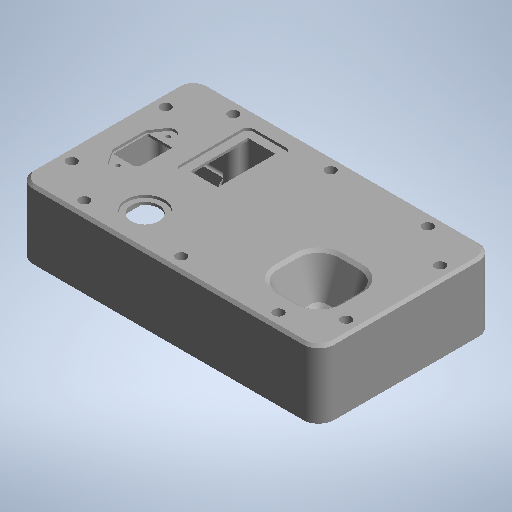
# Autodesk Inventor part: RT_ELE_MC_021_ExtPowerFilterCaseTop
Saved by Autodesk Inventor 2025.4 (Build 294407000, 407)
## iProperties
Created: 2026-08-13
Part Number: RT_ELE_MC_021_ExtPowerFilterCaseTop
Material: Générique
Document SubType Name: Modeling
Designer: louis
Density: 1 g/cm^3
Appearance: Par défaut
Author: louis
Autodesk Inventor part; units mm, degrees
ref_plane "YZ Plane" through (0, 0, 0) normal (1, 0, 0) x (0, 1, 0)
ref_plane "XZ Plane" through (0, 0, 0) normal (0, 1, 0) x (-1, 0, 0)
sketch "Sketch2" plane through (0, 0, 0) normal (0, 0, 1) x (1, 0, 0)
  line L0 (-120, -70) -> (120, -70)
  line L1 (120, -70) -> (120, 70)
  line L2 (120, 70) -> (-120, 70)
  line L3 (-120, 70) -> (-120, -70)
  line L4 (-120, -70) -> (120, 70) construction
  line L5 (120, -70) -> (-120, 70) construction
  line L6 (-112.5, 62.5) -> (112.5, 62.5)
  line L7 (112.5, 62.5) -> (112.5, -62.5)
  line L8 (112.5, -62.5) -> (-112.5, -62.5)
  line L9 (-112.5, -62.5) -> (-112.5, 62.5)
  line L10 (-110, -17.5) -> (110, -17.5) construction
  line L11 (110, -17.5) -> (110, 17.5) construction
  line L12 (110, 17.5) -> (-110, 17.5) construction
  line L13 (-110, 17.5) -> (-110, -17.5) construction
  line L14 (-110, -17.5) -> (110, 17.5) construction
  line L15 (110, -17.5) -> (-110, 17.5) construction
  line L16 (-10, 50) -> (100, 50) construction
  line L17 (100, 50) -> (100, -50) construction
  line L18 (100, -50) -> (-10, -50) construction
  line L19 (-10, -50) -> (-10, 50) construction
  line L20 (-10, 50) -> (100, -50) construction
  line L21 (-10, -50) -> (100, 50) construction
  line L22 (0, 0) -> (110, 0) construction
  circle A0 centre (-109.5, 37.5) radius 2.8
  circle A1 centre (77.5, 59.5) radius 2.8
  circle A2 centre (-77.5, 59.5) radius 2.8
  circle A3 centre (-109.5, -37.5) radius 2.8
  circle A4 centre (-77.5, -59.5) radius 2.8
  circle A5 centre (109.5, 37.5) radius 2.8
  circle A6 centre (109.5, -37.5) radius 2.8
  circle A7 centre (77.5, -59.5) radius 2.8
  line L23 (0, 0) -> (0, 62.5) construction
  circle A8 centre (0, 59.5) radius 2.8
  circle A9 centre (0, -59.5) radius 2.8
  circle A10 centre (-77.5, 59.5) radius 6
  circle A11 centre (77.5, 59.5) radius 6
  circle A12 centre (0, 59.5) radius 6
  circle A13 centre (-109.5, 37.5) radius 6
  circle A14 centre (109.5, 37.5) radius 6
  circle A15 centre (-109.5, -37.5) radius 6
  circle A16 centre (-77.5, -59.5) radius 6
  circle A17 centre (0, -59.5) radius 6
  circle A18 centre (77.5, -59.5) radius 6
  circle A19 centre (109.5, -37.5) radius 6
  point P0 (100, 0)
  point P1 (-112.5, 42.6962)
  point P2 (-82.6962, 62.5)
  point P3 (-72.3038, 62.5)
  point P4 (-5.1962, 62.5)
  point P5 (5.1962, 62.5)
  point P6 (72.3038, 62.5)
  point P7 (82.6962, 62.5)
  point P8 (112.5, 42.6962)
  point P9 (112.5, 32.3038)
  point P10 (112.5, -32.3038)
  point P11 (112.5, -42.6962)
  point P12 (82.6962, -62.5)
  point P13 (72.3038, -62.5)
  point P14 (5.1962, -62.5)
  point P15 (-5.1962, -62.5)
  point P16 (-72.3038, -62.5)
  point P17 (-82.6962, -62.5)
  point P18 (-112.5, -42.6962)
  point P19 (-112.5, -32.3038)
  point P20 (-112.5, 32.3038)
  dimension "d0" = 240
  dimension "d1" = 140
  dimension "d2" = 7.5
  dimension "d3" = 220
  dimension "d4" = 35
  dimension "d5" = 110
  dimension "d6" = 100
  dimension "d7" = 10
  dimension "d8" = 5.6
  dimension "d9" = 5.6
  dimension "d10" = 3
  dimension "d11" = 3
  dimension "d12" = 5.6
  dimension "d13" = 3
  dimension "d14" = 25
  dimension "d15" = 35
  dimension "d16" = 12
  dimension "d17" = 12
  dimension "d18" = 12
  dimension "d19" = 12
  dimension "d20" = 12
  constraints: 48 end point, 20 centre point, 8 parallel, 7 midpoint, 5 coincident, 5 symmetric about line, 4 perpendicular, 3 horizontal, 2 point on line, 15 other
  measures "d0" distance of L5.end L4.end
  measures "d1" distance of L4.end L0.end
  measures "d2" distance between parallel lines of L2 L6
  measures "d3" distance of L15.end L12.start
  measures "d4" distance of L12.start L15.start
  measures "d5" distance of L20.end L19.start
  measures "d6" distance of L16.end L20.end
  measures "d7" distance from line of point (100, 0) L11
  measures "d8" diameter of A0
  measures "d9" diameter of A2
  measures "d10" distance from line of L6 A2.centre
  measures "d11" distance from line of L9 A0.centre
  measures "d12" diameter of A8
  measures "d13" distance from line of L6 A8.centre
  measures "d14" distance from line of L6 A0.centre
  measures "d15" distance from line of L9 A2.centre
  measures "d16" diameter of A13
  measures "d17" diameter of A10
  measures "d18" diameter of A11
  measures "d19" diameter of A12
  measures "d20" diameter of A14
extrude "Extrusion2" add sketch "Sketch2" against normal blind 4 contours L3 L2 L1 L0 | L6 A10 A12 A11 L7 A14 A19 L8 A18 A17 A16 L9 A15 A13 | A10 L6 | L6 A10 | A13 L9 | L9 A13 | A12 L6 | L6 A12 | A15 L9 | L9 A15 | A11 L6 | L6 A11 | A16 L8 | L8 A16 | A14 L7 | L7 A14 | A17 L8 | L8 A17 | A19 L7 | L7 A19 | A18 L8 | L8 A18 | A0 | A1 | A2 | A3 | A4 | A5 | A6 | A7 | A8 | A9
extrude "Extrusion1" add sketch "Sketch2" against normal blind 54 contours L3 L2 L1 L0 | A10 L6 | L6 A10 | A13 L9 | L9 A13 | A12 L6 | L6 A12 | A15 L9 | L9 A15 | A11 L6 | L6 A11 | A16 L8 | L8 A16 | A14 L7 | L7 A14 | A17 L8 | L8 A17 | A19 L7 | L7 A19 | A18 L8 | L8 A18 | A0 | A1 | A2 | A3 | A4 | A5 | A6 | A7 | A8 | A9
fillet "Fillet2" radius 12.5 4 edges at (-120, 70, -27) (120, 70, -27) (-120, -70, -27) (120, -70, -27)
fillet "Fillet3" radius 5 4 edges at (-112.5, 62.5, -29) (-112.5, -62.5, -29) (112.5, 62.5, -29) (112.5, -62.5, -29)
chamfer "Chamfer1" distance 2 angle 45 26 edges at (-38.75, -62.5, -4) (-95.0981, -62.5, -4) (-111.0355, -61.0355, -4) (-112.5, -50.0981, -4) (-112.5, 0, -4) (38.75, -62.5, -4) (95.0981, -62.5, -4) (111.0355, -61.0355, -4) (112.5, -50.0981, -4) (112.5, 0, -4) (95.0981, 62.5, -4) (111.0355, 61.0355, -4) (112.5, 50.0981, -4) (38.75, 62.5, -4) (-38.75, 62.5, -4) (-95.0981, 62.5, -4) (-111.0355, 61.0355, -4) (-112.5, 50.0981, -4) (0, 70, 0) (-116.3388, 66.3388, 0) (-120, 0, 0) (-116.3388, -66.3388, 0) (0, -70, 0) (116.3388, -66.3388, 0) (120, 0, 0) (116.3388, 66.3388, 0)
fillet "Fillet1" radius 5 30 edges at (-112.5, -42.6962, -30) (-82.6962, -62.5, -30) (-72.3038, -62.5, -30) (-5.1962, -62.5, -30) (5.1962, -62.5, -30) (72.3038, -62.5, -30) (82.6962, -62.5, -30) (112.5, -42.6962, -30) (112.5, -32.3038, -30) (112.5, 32.3038, -30) (112.5, 42.6962, -30) (82.6962, 62.5, -30) (72.3038, 62.5, -30) (5.1962, 62.5, -30) (-5.1962, 62.5, -30) (-72.3038, 62.5, -30) (-82.6962, 62.5, -30) (-112.5, 32.3038, -30) (-112.5, 42.6962, -30) (-112.5, -32.3038, -30) (-77.5, -53.5, -4) (-103.5, -37.5, -4) (0, 53.5, -4) (-77.5, 53.5, -4) (103.5, 37.5, -4) (77.5, 53.5, -4) (-103.5, 37.5, -4) (0, -53.5, -4) (77.5, -53.5, -4) (103.5, -37.5, -4)
hole "Hole1" at (77.5, -59.5, 0) at (109.5, -37.5, 0) at (109.5, 37.5, 0) at (77.5, 59.5, 0) at (0, 59.5, 0) at (-77.5, 59.5, 0) at (-109.5, 37.5, 0) at (-109.5, -37.5, 0) at (-77.5, -59.5, 0) at (0, -59.5, 0) direction (0, 0, -1) diameter 4.5 end through all counterbore diameter 8 counterbore depth 44 clearance for "Socket Head Cap Screw" size "M4" standard "Ansi Metric M Profile"
sketch "Sketch3" plane through (0, 0, 0) normal (0, 0, 1) x (1, 0, 0)
  line L0 (-35.25, 50.8) -> (-57.25, 50.8)
  line L1 (-57.25, 50.8) -> (-57.25, 4.8)
  line L2 (-57.25, 4.8) -> (-35.25, 4.8)
  line L3 (-35.25, 4.8) -> (-35.25, 50.8)
  line L4 (-35.25, 50.8) -> (-57.25, 4.8) construction
  line L5 (-57.25, 50.8) -> (-35.25, 4.8) construction
  line L6 (-33.75, -1.7) -> (-58.75, -1.7)
  line L7 (-63.75, 3.3) -> (-63.75, 52.3)
  line L8 (-58.75, 57.3) -> (-33.75, 57.3)
  line L9 (-28.75, 52.3) -> (-28.75, 3.3)
  arc A0 (-33.75, -1.7) -> (-28.75, 3.3) centre (-33.75, 3.3) ccw
  arc A1 (-28.75, 52.3) -> (-33.75, 57.3) centre (-33.75, 52.3) ccw
  arc A2 (-58.75, 57.3) -> (-63.75, 52.3) centre (-58.75, 52.3) ccw
  arc A3 (-63.75, 3.3) -> (-58.75, -1.7) centre (-58.75, 3.3) ccw
  circle A4 centre (-90, 20) radius 5.6
  circle A5 centre (-90, -20) radius 5.6
  line L10 (-101.25, -12.25) -> (-101.25, 12.25)
  line L11 (-98.25, 15.25) -> (-81.75, 15.25)
  line L12 (-78.75, 12.25) -> (-78.75, -12.25)
  line L13 (-81.75, -15.25) -> (-98.25, -15.25)
  line L14 (-101.25, -15.25) -> (-78.75, 15.25) construction
  line L15 (-101.25, 15.25) -> (-78.75, -15.25) construction
  line L16 (-109.6425, -25.6) -> (-109.6425, 25.6) construction
  line L17 (-109.6425, 25.6) -> (-70.3575, 25.6) construction
  line L18 (-70.3575, 25.6) -> (-70.3575, -25.6) construction
  line L19 (-70.3575, -25.6) -> (-109.6425, -25.6) construction
  line L20 (-109.6425, -25.6) -> (-70.3575, 25.6) construction
  line L21 (-109.6425, 25.6) -> (-70.3575, -25.6) construction
  line L22 (-90, 20) -> (-90, 0) construction
  arc A6 (-78.75, 12.25) -> (-81.75, 15.25) centre (-81.75, 12.25) ccw
  arc A7 (-81.75, -15.25) -> (-78.75, -12.25) centre (-81.75, -12.25) ccw
  arc A8 (-101.25, -12.25) -> (-98.25, -15.25) centre (-98.25, -12.25) ccw
  arc A9 (-98.25, 15.25) -> (-101.25, 12.25) centre (-98.25, 12.25) ccw
  line L23 (-85.3308, 23.0917) -> (-79.2487, 13.9063)
  line L24 (-94.6692, 23.0917) -> (-100.7513, 13.9063)
  line L25 (-94.6692, -23.0917) -> (-100.7513, -13.9063)
  line L26 (-79.2487, -13.9063) -> (-85.3308, -23.0917)
  line L27 (-90, 0) -> (-90, -20) construction
  line L28 (-100, -14) -> (-100, 14)
  line L29 (-100, 14) -> (-80, 14)
  line L30 (-80, 14) -> (-80, -14)
  line L31 (-80, -14) -> (-100, -14)
  line L32 (-100, -14) -> (-80, 14) construction
  line L33 (-100, 14) -> (-80, -14) construction
  circle A10 centre (-46.25, -42.2) radius 11
  circle A11 centre (-46.25, -42.2) radius 15.1
  line L34 (-46.25, 27.8) -> (-46.25, -42.2) construction
  line L35 (-101.25, 57.3) -> (-28.75, 57.3)
  line L36 (-28.75, 57.3) -> (-28.75, -57.3)
  line L37 (-28.75, -57.3) -> (-101.25, -57.3)
  line L38 (-101.25, -57.3) -> (-101.25, 57.3)
  line L39 (-101.25, 57.3) -> (-28.75, -57.3) construction
  line L40 (-28.75, 57.3) -> (-101.25, -57.3) construction
  line L41 (-65, 0) -> (-90, 0) construction
  line L42 (0, 0) -> (-65, 0) construction
  point P0 (-28.75, -1.7)
  point P1 (-63.75, -1.7)
  dimension "d38" = 22
  dimension "d39" = 46
  dimension "d40" = 35
  dimension "d41" = 5
  dimension "d42" = 22.5
  dimension "d43" = 30.5
  dimension "d45" = 51.2
  dimension "d46" = 3
  dimension "d47" = 28
  dimension "d48" = 20
  dimension "d49" = 22
  dimension "d50" = 30.2
  dimension "d51" = 70
  dimension "d54" = 40
  dimension "d55" = 25
  dimension "d56" = 65
  constraints: 86 end point, 27 tangent, 24 point on circle, 14 parallel, 12 centre point, 12 point on line, 10 midpoint, 7 equal radius, 7 perpendicular, 4 collinear, 4 horizontal, 1 coincident, 1 vertical, 3 other
  measures "d38" distance of L2.end L1.end
  measures "d39" distance of L1.end L0.end
  measures "d40" distance of point (-28.75, -1.7) point (-63.75, -1.7)
  measures "d41" radius of A0
  measures "d42" distance of L15.end L14.start
  measures "d43" distance of L14.end L15.end
  measures "d45" distance of L17.end L18.end
  measures "d46" radius of A6
  measures "d47" distance of L29.end L30.end
  measures "d48" distance of L28.end L29.end
  measures "d49" diameter of A10
  measures "d50" diameter of A11
  measures "d51" distance of L34.start L34.end
  measures "d54" distance of L22.start L27.end
  measures "d55" distance of L41.start L22.end
  measures "d56" distance of L42.start L41.start
extrude "Extrusion3" cut sketch "Sketch3" against normal through all contours L3 L2 L1 L0 | L28 L29 L30 L31 | A10
extrude "Extrusion4" cut sketch "Sketch3" against normal blind 2 contours L3 L2 L1 L0 | A11 | L6 A3 L7 A2 L8 A1 L9 A0 | L10 A9 L11 A4 A6 L12 A7 L13 A5 A8 | A8 L13 A5 L25 | L24 A4 L11 A9 | A5 L13 | A4 L11 | A5 L13 | A5 L13 A7 L26 | L11 A4 | L23 A6 L11 A4 | L28 L29 L30 L31 | A10
hole "Hole2" at (-90, 20, 0) at (-90, -20, 0) direction (0, 0, -1) diameter 3.3 end through all
fillet "Fillet4" radius 1 8 edges at (-57.25, 50.8, -3) (-57.25, 4.8, -3) (-35.25, 4.8, -3) (-35.25, 50.8, -3) (-80, 14, -3) (-100, 14, -3) (-100, -14, -3) (-80, -14, -3)
ref_plane "Work Plane1" through (0, 0, -34) normal (0, 0, -1) x (-1, 0, 0)
sketch "Sketch4" plane through (0, 0, -34) normal (0, 0, -1) x (-1, 0, 0)
  line L0 (-62, -30) -> (-78, -30)
  line L1 (-80, -28) -> (-80, -12)
  line L2 (-78, -10) -> (-62, -10)
  line L3 (-60, -12) -> (-60, -28)
  line L4 (-60, -30) -> (-80, -10) construction
  line L5 (-80, -30) -> (-60, -10) construction
  line L6 (-82.5, 0) -> (-57.5, 0)
  line L7 (-50, -7.5) -> (-50, -32.5)
  line L8 (-57.5, -40) -> (-82.5, -40)
  line L9 (-90, -32.5) -> (-90, -7.5)
  line L10 (-90, 0) -> (-50, -40) construction
  line L11 (-50, 0) -> (-90, -40) construction
  arc A0 (-62, -30) -> (-60, -28) centre (-62, -28) ccw
  arc A1 (-60, -12) -> (-62, -10) centre (-62, -12) ccw
  arc A2 (-78, -10) -> (-80, -12) centre (-78, -12) ccw
  arc A3 (-80, -28) -> (-78, -30) centre (-78, -28) ccw
  arc A4 (-57.5, -40) -> (-50, -32.5) centre (-57.5, -32.5) ccw
  arc A5 (-90, -32.5) -> (-82.5, -40) centre (-82.5, -32.5) ccw
  arc A6 (-82.5, 0) -> (-90, -7.5) centre (-82.5, -7.5) ccw
  arc A7 (-50, -7.5) -> (-57.5, 0) centre (-57.5, -7.5) ccw
  line L12 (-112.5, -26.6833) -> (-112.5, 26.6833) projected
  line L13 (-78, -32.5) -> (-62, -32.5)
  arc A8 (-62, -32.5) -> (-57.5, -28) centre (-62, -28) ccw
  line L14 (-57.5, -28) -> (-57.5, -12)
  arc A9 (-57.5, -12) -> (-62, -7.5) centre (-62, -12) ccw
  line L15 (-62, -7.5) -> (-78, -7.5)
  arc A10 (-78, -7.5) -> (-82.5, -12) centre (-78, -12) ccw
  line L16 (-82.5, -12) -> (-82.5, -28)
  arc A11 (-82.5, -28) -> (-78, -32.5) centre (-78, -28) ccw
  point P0 (0, 0)
  point P1 (-70, -20)
  dimension "d70" = 20
  dimension "d71" = 20
  dimension "d72" = 40
  dimension "d73" = 40
  dimension "d74" = 2
  dimension "d75" = 7.5
  dimension "d76" = 20
  dimension "d77" = 70
  dimension "d78" = 22.5
  dimension "d89" = 2.5
  constraints: 32 end point, 24 point on circle, 16 point on line, 16 tangent, 12 centre point, 6 equal radius, 6 parallel, 4 midpoint, 3 perpendicular, 2 horizontal, 7 other
  measures "d70" distance of L4.end L5.end
  measures "d71" distance of L5.start L4.end
  measures "d72" distance of L10.end L11.end
  measures "d73" distance of L11.start L10.end
  measures "d74" radius of A0
  measures "d75" radius of A4
  measures "d76" vertical distance of point (0, 0) point (-70, -20)
  measures "d77" horizontal distance of point (-70, -20) point (0, 0)
  measures "d78" distance between parallel lines of L12 L9
  measures "d89" distance between parallel lines of L0 L13
sketch "Sketch5" plane through (0, 0, 0) normal (0, 0, 1) x (1, 0, 0)
  line L0 (62, -30) -> (78, -30) construction
  line L1 (78, -10) -> (62, -10) construction
  line L2 (60, -30) -> (80, -10) construction
  line L3 (80, -30) -> (60, -10) construction
  line L4 (57.5, -40) -> (82.5, -40) construction
  line L5 (82.5, 0) -> (57.5, 0) construction
  line L6 (50, 0) -> (90, -40) construction
  arc A0 (62, -10) -> (60, -12) centre (62, -12) ccw construction
  line L7 (50, -7.5) -> (50, -32.5) construction
  arc A1 (57.5, 0) -> (50, -7.5) centre (57.5, -7.5) ccw construction
  line L8 (60, -12) -> (60, -28) construction
  arc A2 (80, -12) -> (78, -10) centre (78, -12) ccw construction
  arc A3 (78, -30) -> (80, -28) centre (78, -28) ccw construction
  line L9 (80, -28) -> (80, -12) construction
  arc A4 (82.5, -40) -> (90, -32.5) centre (82.5, -32.5) ccw construction
  line L10 (90, -32.5) -> (90, -7.5) construction
  arc A5 (90, -7.5) -> (82.5, 0) centre (82.5, -7.5) ccw construction
  arc A6 (50, -32.5) -> (57.5, -40) centre (57.5, -32.5) ccw construction
  arc A7 (60, -28) -> (62, -30) centre (62, -28) ccw construction
  line L11 (37.5, -7.5) -> (37.5, -32.5)
  arc A8 (37.5, -32.5) -> (57.5, -52.5) centre (57.5, -32.5) ccw
  line L12 (57.5, -52.5) -> (82.5, -52.5)
  arc A9 (82.5, -52.5) -> (102.5, -32.5) centre (82.5, -32.5) ccw
  line L13 (102.5, -32.5) -> (102.5, -7.5)
  arc A10 (102.5, -7.5) -> (82.5, 12.5) centre (82.5, -7.5) ccw
  line L14 (82.5, 12.5) -> (57.5, 12.5)
  arc A11 (57.5, 12.5) -> (37.5, -7.5) centre (57.5, -7.5) ccw
  line L15 (47.5, -28) -> (47.5, -12)
  arc A12 (62, 2.5) -> (47.5, -12) centre (62, -12) ccw
  line L16 (62, 2.5) -> (78, 2.5)
  arc A13 (92.5, -12) -> (78, 2.5) centre (78, -12) ccw
  line L17 (92.5, -12) -> (92.5, -28)
  arc A14 (78, -42.5) -> (92.5, -28) centre (78, -28) ccw
  line L18 (78, -42.5) -> (62, -42.5)
  arc A15 (47.5, -28) -> (62, -42.5) centre (62, -28) ccw
  line L19 (62, -45) -> (78, -45)
  arc A16 (78, -45) -> (95, -28) centre (78, -28) ccw
  line L20 (95, -28) -> (95, -12)
  arc A17 (95, -12) -> (78, 5) centre (78, -12) ccw
  line L21 (78, 5) -> (62, 5)
  arc A18 (62, 5) -> (45, -12) centre (62, -12) ccw
  line L22 (45, -12) -> (45, -28)
  arc A19 (45, -28) -> (62, -45) centre (62, -28) ccw
  point P0 (0, 0)
  point P1 (70, -20)
  point P2 (50, -40)
  dimension "d79" = 12.5
  dimension "d80" = 12.5
  dimension "d90" = 2.5
  constraints: 24 end point, 24 point on circle, 12 centre point, 21 other
  measures "d79" radial gap between concentric circles of A1 A11
  measures "d80" distance between parallel lines of L8 L15
  measures "d90" distance between parallel lines of L18 L19
loft "Loft1" add profiles "Sketch4", "Sketch5" contours L0 A3 L1 A2 L2 A1 L3 A0 | L6 A7 L7 A4 L8 A5 L9 A6 | A11 L16 A10 L15 A9 L14 A8 L13 / A11 L14 A10 L13 A9 L12 A8 L11 | L15 A12 L16 A13 L17 A14 L18 A15 | A19 L22 A18 L21 A17 L20 A16 L19
loft "Loft2" cut profiles "Sketch4", "Sketch5" contours L0 A3 L1 A2 L2 A1 L3 A0 | A11 L16 A10 L15 A9 L14 A8 L13 / L15 A12 L16 A13 L17 A14 L18 A15 | A19 L22 A18 L21 A17 L20 A16 L19
extrude "Extrusion5" add sketch "Sketch4" against normal blind 2 contours L6 A7 L7 A4 L8 A5 L9 A6 | A11 L16 A10 L15 A9 L14 A8 L13
chamfer "Chamfer2" distance 3.2 angle 45 8 edges at (58.2981, -8.2981, -32) (70, -6.7647, -32) (81.7019, -8.2981, -32) (83.2353, -20, -32) (81.7019, -31.7019, -32) (70, -33.2353, -32) (58.2981, -31.7019, -32) (56.7647, -20, -32)
chamfer "Chamfer3" distance 2 angle 45 8 edges at (49.9792, 0.0208, 0) (70, 5, 0) (90.0208, 0.0208, 0) (95, -20, 0) (90.0208, -40.0208, 0) (70, -45, 0) (49.9792, -40.0208, 0) (45, -20, 0)
chamfer "Chamfer4" distance 1 angle 45 10 edges at (77.5, 63.5, -44) (109.5, 41.5, -44) (0, 63.5, -44) (-77.5, 63.5, -44) (-109.5, 41.5, -44) (-109.5, -33.5, -44) (-77.5, -55.5, -44) (0, -55.5, -44) (77.5, -55.5, -44) (109.5, -33.5, -44)
sketch "Sketch6" plane through (0, 0, -54) normal (0, 0, -1) x (-1, 0, 0)
  circle A0 centre (0, -59.5) radius 2.25 projected
  circle A1 centre (77.5, -59.5) radius 2.25 projected
  circle A2 centre (109.5, -37.5) radius 2.25 projected
  circle A3 centre (109.5, 37.5) radius 2.25 projected
  circle A4 centre (77.5, 59.5) radius 2.25 projected
  circle A5 centre (0, 59.5) radius 2.25 projected
  circle A6 centre (-77.5, 59.5) radius 2.25 projected
  circle A7 centre (-109.5, 37.5) radius 2.25 projected
  circle A8 centre (-109.5, -37.5) radius 2.25 projected
  circle A9 centre (-77.5, -59.5) radius 2.25 projected
  arc A10 (-120, -57.5) -> (-107.5, -70) centre (-107.5, -57.5) ccw projected
  line L0 (-107.5, -70) -> (107.5, -70) projected
  arc A11 (107.5, -70) -> (120, -57.5) centre (107.5, -57.5) ccw projected
  line L1 (120, -57.5) -> (120, 57.5) projected
  arc A12 (120, 57.5) -> (107.5, 70) centre (107.5, 57.5) ccw projected
  line L2 (107.5, 70) -> (-107.5, 70) projected
  arc A13 (-107.5, 70) -> (-120, 57.5) centre (-107.5, 57.5) ccw projected
  line L3 (-120, 57.5) -> (-120, -57.5) projected
  arc A14 (108.4091, 43.4) -> (108.4091, 31.6) centre (109.5, 37.5) ccw projected
  arc A15 (112.5, 26.6833) -> (108.4091, 31.6) centre (107.5, 26.6833) ccw projected
  line L4 (112.5, 26.6833) -> (112.5, -26.6833) projected
  arc A16 (108.4091, -31.6) -> (112.5, -26.6833) centre (107.5, -26.6833) ccw projected
  arc A17 (108.4091, -31.6) -> (108.4091, -43.4) centre (109.5, -37.5) ccw projected
  arc A18 (112.5, -48.3167) -> (108.4091, -43.4) centre (107.5, -48.3167) ccw projected
  line L5 (112.5, -48.3167) -> (112.5, -57.5) projected
  arc A19 (107.5, -62.5) -> (112.5, -57.5) centre (107.5, -57.5) ccw projected
  line L6 (107.5, -62.5) -> (88.3167, -62.5) projected
  arc A20 (83.4, -58.4091) -> (88.3167, -62.5) centre (88.3167, -57.5) ccw projected
  arc A21 (83.4, -58.4091) -> (71.6, -58.4091) centre (77.5, -59.5) ccw projected
  arc A22 (66.6833, -62.5) -> (71.6, -58.4091) centre (66.6833, -57.5) ccw projected
  line L7 (66.6833, -62.5) -> (10.8167, -62.5) projected
  arc A23 (5.9, -58.4091) -> (10.8167, -62.5) centre (10.8167, -57.5) ccw projected
  arc A24 (5.9, -58.4091) -> (-5.9, -58.4091) centre (0, -59.5) ccw projected
  arc A25 (-10.8167, -62.5) -> (-5.9, -58.4091) centre (-10.8167, -57.5) ccw projected
  line L8 (-10.8167, -62.5) -> (-66.6833, -62.5) projected
  arc A26 (-71.6, -58.4091) -> (-66.6833, -62.5) centre (-66.6833, -57.5) ccw projected
  arc A27 (-71.6, -58.4091) -> (-83.4, -58.4091) centre (-77.5, -59.5) ccw projected
  arc A28 (-88.3167, -62.5) -> (-83.4, -58.4091) centre (-88.3167, -57.5) ccw projected
  line L9 (-88.3167, -62.5) -> (-107.5, -62.5) projected
  arc A29 (-112.5, -57.5) -> (-107.5, -62.5) centre (-107.5, -57.5) ccw projected
  line L10 (-112.5, -57.5) -> (-112.5, -48.3167) projected
  arc A30 (-108.4091, -43.4) -> (-112.5, -48.3167) centre (-107.5, -48.3167) ccw projected
  arc A31 (-108.4091, -43.4) -> (-108.4091, -31.6) centre (-109.5, -37.5) ccw projected
  arc A32 (-112.5, -26.6833) -> (-108.4091, -31.6) centre (-107.5, -26.6833) ccw projected
  line L11 (-112.5, -26.6833) -> (-112.5, 26.6833) projected
  arc A33 (-108.4091, 31.6) -> (-112.5, 26.6833) centre (-107.5, 26.6833) ccw projected
  arc A34 (-108.4091, 31.6) -> (-108.4091, 43.4) centre (-109.5, 37.5) ccw projected
  arc A35 (-112.5, 48.3167) -> (-108.4091, 43.4) centre (-107.5, 48.3167) ccw projected
  line L12 (-112.5, 48.3167) -> (-112.5, 57.5) projected
  arc A36 (-107.5, 62.5) -> (-112.5, 57.5) centre (-107.5, 57.5) ccw projected
  line L13 (-107.5, 62.5) -> (-88.3167, 62.5) projected
  arc A37 (-83.4, 58.4091) -> (-88.3167, 62.5) centre (-88.3167, 57.5) ccw projected
  arc A38 (-83.4, 58.4091) -> (-71.6, 58.4091) centre (-77.5, 59.5) ccw projected
  arc A39 (-66.6833, 62.5) -> (-71.6, 58.4091) centre (-66.6833, 57.5) ccw projected
  line L14 (-66.6833, 62.5) -> (-10.8167, 62.5) projected
  arc A40 (-5.9, 58.4091) -> (-10.8167, 62.5) centre (-10.8167, 57.5) ccw projected
  arc A41 (-5.9, 58.4091) -> (5.9, 58.4091) centre (0, 59.5) ccw projected
  arc A42 (10.8167, 62.5) -> (5.9, 58.4091) centre (10.8167, 57.5) ccw projected
  line L15 (10.8167, 62.5) -> (66.6833, 62.5) projected
  arc A43 (71.6, 58.4091) -> (66.6833, 62.5) centre (66.6833, 57.5) ccw projected
  arc A44 (71.6, 58.4091) -> (83.4, 58.4091) centre (77.5, 59.5) ccw projected
  arc A45 (88.3167, 62.5) -> (83.4, 58.4091) centre (88.3167, 57.5) ccw projected
  line L16 (88.3167, 62.5) -> (107.5, 62.5) projected
  arc A46 (112.5, 57.5) -> (107.5, 62.5) centre (107.5, 57.5) ccw projected
  line L17 (112.5, 57.5) -> (112.5, 48.3167) projected
  arc A47 (108.4091, 43.4) -> (112.5, 48.3167) centre (107.5, 48.3167) ccw projected
  arc A48 (-69.6333, -58.0455) -> (-85.3667, -58.0455) centre (-77.5, -59.5) ccw
  arc A49 (-69.6333, -58.0455) -> (-66.6833, -60.5) centre (-66.6833, -57.5) ccw
  line L18 (-66.6833, -60.5) -> (-10.8167, -60.5)
  arc A50 (-10.8167, -60.5) -> (-7.8667, -58.0455) centre (-10.8167, -57.5) ccw
  arc A51 (7.8667, -58.0455) -> (-7.8667, -58.0455) centre (0, -59.5) ccw
  arc A52 (7.8667, -58.0455) -> (10.8167, -60.5) centre (10.8167, -57.5) ccw
  line L19 (10.8167, -60.5) -> (66.6833, -60.5)
  arc A53 (66.6833, -60.5) -> (69.6333, -58.0455) centre (66.6833, -57.5) ccw
  arc A54 (85.3667, -58.0455) -> (69.6333, -58.0455) centre (77.5, -59.5) ccw
  arc A55 (85.3667, -58.0455) -> (88.3167, -60.5) centre (88.3167, -57.5) ccw
  line L20 (88.3167, -60.5) -> (107.5, -60.5)
  arc A56 (107.5, -60.5) -> (110.5, -57.5) centre (107.5, -57.5) ccw
  line L21 (110.5, -57.5) -> (110.5, -48.3167)
  arc A57 (110.5, -48.3167) -> (108.0455, -45.3667) centre (107.5, -48.3167) ccw
  arc A58 (108.0455, -29.6333) -> (108.0455, -45.3667) centre (109.5, -37.5) ccw
  arc A59 (108.0455, -29.6333) -> (110.5, -26.6833) centre (107.5, -26.6833) ccw
  line L22 (110.5, -26.6833) -> (110.5, 26.6833)
  arc A60 (110.5, 26.6833) -> (108.0455, 29.6333) centre (107.5, 26.6833) ccw
  arc A61 (108.0455, 45.3667) -> (108.0455, 29.6333) centre (109.5, 37.5) ccw
  arc A62 (108.0455, 45.3667) -> (110.5, 48.3167) centre (107.5, 48.3167) ccw
  line L23 (110.5, 48.3167) -> (110.5, 57.5)
  arc A63 (110.5, 57.5) -> (107.5, 60.5) centre (107.5, 57.5) ccw
  line L24 (107.5, 60.5) -> (88.3167, 60.5)
  arc A64 (88.3167, 60.5) -> (85.3667, 58.0455) centre (88.3167, 57.5) ccw
  arc A65 (69.6333, 58.0455) -> (85.3667, 58.0455) centre (77.5, 59.5) ccw
  arc A66 (69.6333, 58.0455) -> (66.6833, 60.5) centre (66.6833, 57.5) ccw
  line L25 (66.6833, 60.5) -> (10.8167, 60.5)
  arc A67 (10.8167, 60.5) -> (7.8667, 58.0455) centre (10.8167, 57.5) ccw
  arc A68 (-7.8667, 58.0455) -> (7.8667, 58.0455) centre (0, 59.5) ccw
  arc A69 (-7.8667, 58.0455) -> (-10.8167, 60.5) centre (-10.8167, 57.5) ccw
  line L26 (-10.8167, 60.5) -> (-66.6833, 60.5)
  arc A70 (-66.6833, 60.5) -> (-69.6333, 58.0455) centre (-66.6833, 57.5) ccw
  arc A71 (-85.3667, 58.0455) -> (-69.6333, 58.0455) centre (-77.5, 59.5) ccw
  arc A72 (-85.3667, 58.0455) -> (-88.3167, 60.5) centre (-88.3167, 57.5) ccw
  line L27 (-88.3167, 60.5) -> (-107.5, 60.5)
  arc A73 (-107.5, 60.5) -> (-110.5, 57.5) centre (-107.5, 57.5) ccw
  line L28 (-110.5, 57.5) -> (-110.5, 48.3167)
  arc A74 (-110.5, 48.3167) -> (-108.0455, 45.3667) centre (-107.5, 48.3167) ccw
  arc A75 (-108.0455, 29.6333) -> (-108.0455, 45.3667) centre (-109.5, 37.5) ccw
  arc A76 (-108.0455, 29.6333) -> (-110.5, 26.6833) centre (-107.5, 26.6833) ccw
  line L29 (-110.5, 26.6833) -> (-110.5, -26.6833)
  arc A77 (-110.5, -26.6833) -> (-108.0455, -29.6333) centre (-107.5, -26.6833) ccw
  arc A78 (-108.0455, -45.3667) -> (-108.0455, -29.6333) centre (-109.5, -37.5) ccw
  arc A79 (-108.0455, -45.3667) -> (-110.5, -48.3167) centre (-107.5, -48.3167) ccw
  line L30 (-110.5, -48.3167) -> (-110.5, -57.5)
  arc A80 (-110.5, -57.5) -> (-107.5, -60.5) centre (-107.5, -57.5) ccw
  line L31 (-107.5, -60.5) -> (-88.3167, -60.5)
  arc A81 (-88.3167, -60.5) -> (-85.3667, -58.0455) centre (-88.3167, -57.5) ccw
  point P0 (0, 0)
  dimension "d102" = 2
  constraints: 68 point on circle, 34 centre point, 28 end point, 47 other
  measures "d102" radial gap between concentric circles of A27 A48
extrude "Extrusion6" add sketch "Sketch6" along normal mid plane 10 contours A14 A15 L4 A16 A17 A18 L5 A19 L6 A20 A21 A22 L7 A23 A24 A25 L8 A26 A27 A28 L9 A29 L10 A30 A31 A32 L11 A33 A34 A35 L12 A36 L13 A37 A38 A39 L14 A40 A41 A42 L15 A43 A44 A45 L16 A46 L17 A47
fillet "Fillet5" radius 2 48 edges at (111.3435, -29.8814, -49) (103.5, -37.5, -49) (111.3435, -45.1186, -49) (112.5, -52.9083, -49) (111.0355, -61.0355, -49) (97.9083, -62.5, -49) (85.1186, -61.3435, -49) (77.5, -53.5, -49) (69.8814, -61.3435, -49) (38.75, -62.5, -49) (7.6186, -61.3435, -49) (0, -53.5, -49) (-7.6186, -61.3435, -49) (-38.75, -62.5, -49) (-69.8814, -61.3435, -49) (-77.5, -53.5, -49) (-85.1186, -61.3435, -49) (-97.9083, -62.5, -49) (-111.0355, -61.0355, -49) (-112.5, -52.9083, -49) (-111.3435, -45.1186, -49) (-103.5, -37.5, -49) (-111.3435, -29.8814, -49) (-112.5, 0, -49) (-111.3435, 29.8814, -49) (-103.5, 37.5, -49) (-111.3435, 45.1186, -49) (-112.5, 52.9083, -49) (-111.0355, 61.0355, -49) (-97.9083, 62.5, -49) (-85.1186, 61.3435, -49) (-77.5, 53.5, -49) (-69.8814, 61.3435, -49) (-38.75, 62.5, -49) (-7.6186, 61.3435, -49) (0, 53.5, -49) (7.6186, 61.3435, -49) (38.75, 62.5, -49) (69.8814, 61.3435, -49) (77.5, 53.5, -49) (85.1186, 61.3435, -49) (97.9083, 62.5, -49) (111.0355, 61.0355, -49) (112.5, 52.9083, -49) (111.3435, 45.1186, -49) (103.5, 37.5, -49) (111.3435, 29.8814, -49) (112.5, 0, -49)
sketch "Sketch7" plane through (0, 0, -59) normal (0, 0, -1) x (-1, 0, 0)
  line L0 (107.5, 62.5) -> (88.3167, 62.5) projected
  arc A0 (88.3167, 62.5) -> (83.4, 58.4091) centre (88.3167, 57.5) ccw projected
  arc A1 (71.6, 58.4091) -> (83.4, 58.4091) centre (77.5, 59.5) ccw projected
  arc A2 (71.6, 58.4091) -> (66.6833, 62.5) centre (66.6833, 57.5) ccw projected
  line L1 (66.6833, 62.5) -> (10.8167, 62.5) projected
  arc A3 (10.8167, 62.5) -> (5.9, 58.4091) centre (10.8167, 57.5) ccw projected
  arc A4 (-5.9, 58.4091) -> (5.9, 58.4091) centre (0, 59.5) ccw projected
  arc A5 (-5.9, 58.4091) -> (-10.8167, 62.5) centre (-10.8167, 57.5) ccw projected
  line L2 (-10.8167, 62.5) -> (-66.6833, 62.5) projected
  arc A6 (-66.6833, 62.5) -> (-71.6, 58.4091) centre (-66.6833, 57.5) ccw projected
  arc A7 (-83.4, 58.4091) -> (-71.6, 58.4091) centre (-77.5, 59.5) ccw projected
  arc A8 (-83.4, 58.4091) -> (-88.3167, 62.5) centre (-88.3167, 57.5) ccw projected
  line L3 (-88.3167, 62.5) -> (-107.5, 62.5) projected
  arc A9 (-107.5, 62.5) -> (-112.5, 57.5) centre (-107.5, 57.5) ccw projected
  line L4 (-112.5, 57.5) -> (-112.5, 48.3167) projected
  arc A10 (-112.5, 48.3167) -> (-108.4091, 43.4) centre (-107.5, 48.3167) ccw projected
  arc A11 (-108.4091, 31.6) -> (-108.4091, 43.4) centre (-109.5, 37.5) ccw projected
  arc A12 (-108.4091, 31.6) -> (-112.5, 26.6833) centre (-107.5, 26.6833) ccw projected
  line L5 (-112.5, 26.6833) -> (-112.5, -26.6833) projected
  arc A13 (-112.5, -26.6833) -> (-108.4091, -31.6) centre (-107.5, -26.6833) ccw projected
  arc A14 (-108.4091, -43.4) -> (-108.4091, -31.6) centre (-109.5, -37.5) ccw projected
  arc A15 (-108.4091, -43.4) -> (-112.5, -48.3167) centre (-107.5, -48.3167) ccw projected
  line L6 (-112.5, -48.3167) -> (-112.5, -57.5) projected
  arc A16 (-112.5, -57.5) -> (-107.5, -62.5) centre (-107.5, -57.5) ccw projected
  line L7 (-107.5, -62.5) -> (-88.3167, -62.5) projected
  arc A17 (-88.3167, -62.5) -> (-83.4, -58.4091) centre (-88.3167, -57.5) ccw projected
  arc A18 (-71.6, -58.4091) -> (-83.4, -58.4091) centre (-77.5, -59.5) ccw projected
  arc A19 (-71.6, -58.4091) -> (-66.6833, -62.5) centre (-66.6833, -57.5) ccw projected
  line L8 (-66.6833, -62.5) -> (-10.8167, -62.5) projected
  arc A20 (-10.8167, -62.5) -> (-5.9, -58.4091) centre (-10.8167, -57.5) ccw projected
  arc A21 (5.9, -58.4091) -> (-5.9, -58.4091) centre (0, -59.5) ccw projected
  arc A22 (5.9, -58.4091) -> (10.8167, -62.5) centre (10.8167, -57.5) ccw projected
  line L9 (10.8167, -62.5) -> (66.6833, -62.5) projected
  arc A23 (66.6833, -62.5) -> (71.6, -58.4091) centre (66.6833, -57.5) ccw projected
  arc A24 (83.4, -58.4091) -> (71.6, -58.4091) centre (77.5, -59.5) ccw projected
  arc A25 (83.4, -58.4091) -> (88.3167, -62.5) centre (88.3167, -57.5) ccw projected
  line L10 (88.3167, -62.5) -> (107.5, -62.5) projected
  arc A26 (107.5, -62.5) -> (112.5, -57.5) centre (107.5, -57.5) ccw projected
  line L11 (112.5, -57.5) -> (112.5, -48.3167) projected
  arc A27 (112.5, -48.3167) -> (108.4091, -43.4) centre (107.5, -48.3167) ccw projected
  arc A28 (108.4091, -31.6) -> (108.4091, -43.4) centre (109.5, -37.5) ccw projected
  arc A29 (108.4091, -31.6) -> (112.5, -26.6833) centre (107.5, -26.6833) ccw projected
  line L12 (112.5, -26.6833) -> (112.5, 26.6833) projected
  arc A30 (112.5, 26.6833) -> (108.4091, 31.6) centre (107.5, 26.6833) ccw projected
  arc A31 (108.4091, 43.4) -> (108.4091, 31.6) centre (109.5, 37.5) ccw projected
  arc A32 (108.4091, 43.4) -> (112.5, 48.3167) centre (107.5, 48.3167) ccw projected
  line L13 (112.5, 48.3167) -> (112.5, 57.5) projected
  arc A33 (112.5, 57.5) -> (107.5, 62.5) centre (107.5, 57.5) ccw projected
  arc A34 (-69.6333, -58.0455) -> (-66.6833, -60.5) centre (-66.6833, -57.5) ccw projected
  arc A35 (-69.6333, -58.0455) -> (-85.3667, -58.0455) centre (-77.5, -59.5) ccw projected
  arc A36 (-88.3167, -60.5) -> (-85.3667, -58.0455) centre (-88.3167, -57.5) ccw projected
  line L14 (-88.3167, -60.5) -> (-107.5, -60.5) projected
  arc A37 (-110.5, -57.5) -> (-107.5, -60.5) centre (-107.5, -57.5) ccw projected
  line L15 (-110.5, -57.5) -> (-110.5, -48.3167) projected
  arc A38 (-108.0455, -45.3667) -> (-110.5, -48.3167) centre (-107.5, -48.3167) ccw projected
  arc A39 (-108.0455, -45.3667) -> (-108.0455, -29.6333) centre (-109.5, -37.5) ccw projected
  arc A40 (-110.5, -26.6833) -> (-108.0455, -29.6333) centre (-107.5, -26.6833) ccw projected
  line L16 (-110.5, -26.6833) -> (-110.5, 26.6833) projected
  arc A41 (-108.0455, 29.6333) -> (-110.5, 26.6833) centre (-107.5, 26.6833) ccw projected
  arc A42 (-108.0455, 29.6333) -> (-108.0455, 45.3667) centre (-109.5, 37.5) ccw projected
  arc A43 (-110.5, 48.3167) -> (-108.0455, 45.3667) centre (-107.5, 48.3167) ccw projected
  line L17 (-110.5, 48.3167) -> (-110.5, 57.5) projected
  arc A44 (-107.5, 60.5) -> (-110.5, 57.5) centre (-107.5, 57.5) ccw projected
  line L18 (-107.5, 60.5) -> (-88.3167, 60.5) projected
  arc A45 (-85.3667, 58.0455) -> (-88.3167, 60.5) centre (-88.3167, 57.5) ccw projected
  arc A46 (-85.3667, 58.0455) -> (-69.6333, 58.0455) centre (-77.5, 59.5) ccw projected
  arc A47 (-66.6833, 60.5) -> (-69.6333, 58.0455) centre (-66.6833, 57.5) ccw projected
  line L19 (-66.6833, 60.5) -> (-10.8167, 60.5) projected
  arc A48 (-7.8667, 58.0455) -> (-10.8167, 60.5) centre (-10.8167, 57.5) ccw projected
  arc A49 (-7.8667, 58.0455) -> (7.8667, 58.0455) centre (0, 59.5) ccw projected
  arc A50 (10.8167, 60.5) -> (7.8667, 58.0455) centre (10.8167, 57.5) ccw projected
  line L20 (10.8167, 60.5) -> (66.6833, 60.5) projected
  arc A51 (69.6333, 58.0455) -> (66.6833, 60.5) centre (66.6833, 57.5) ccw projected
  arc A52 (69.6333, 58.0455) -> (85.3667, 58.0455) centre (77.5, 59.5) ccw projected
  arc A53 (88.3167, 60.5) -> (85.3667, 58.0455) centre (88.3167, 57.5) ccw projected
  line L21 (88.3167, 60.5) -> (107.5, 60.5) projected
  arc A54 (110.5, 57.5) -> (107.5, 60.5) centre (107.5, 57.5) ccw projected
  line L22 (110.5, 57.5) -> (110.5, 48.3167) projected
  arc A55 (108.0455, 45.3667) -> (110.5, 48.3167) centre (107.5, 48.3167) ccw projected
  arc A56 (108.0455, 45.3667) -> (108.0455, 29.6333) centre (109.5, 37.5) ccw projected
  arc A57 (110.5, 26.6833) -> (108.0455, 29.6333) centre (107.5, 26.6833) ccw projected
  line L23 (110.5, 26.6833) -> (110.5, -26.6833) projected
  arc A58 (108.0455, -29.6333) -> (110.5, -26.6833) centre (107.5, -26.6833) ccw projected
  arc A59 (108.0455, -29.6333) -> (108.0455, -45.3667) centre (109.5, -37.5) ccw projected
  arc A60 (110.5, -48.3167) -> (108.0455, -45.3667) centre (107.5, -48.3167) ccw projected
  line L24 (110.5, -48.3167) -> (110.5, -57.5) projected
  arc A61 (107.5, -60.5) -> (110.5, -57.5) centre (107.5, -57.5) ccw projected
  line L25 (107.5, -60.5) -> (88.3167, -60.5) projected
  arc A62 (85.3667, -58.0455) -> (88.3167, -60.5) centre (88.3167, -57.5) ccw projected
  arc A63 (85.3667, -58.0455) -> (69.6333, -58.0455) centre (77.5, -59.5) ccw projected
  arc A64 (66.6833, -60.5) -> (69.6333, -58.0455) centre (66.6833, -57.5) ccw projected
  line L26 (66.6833, -60.5) -> (10.8167, -60.5) projected
  arc A65 (7.8667, -58.0455) -> (10.8167, -60.5) centre (10.8167, -57.5) ccw projected
  arc A66 (7.8667, -58.0455) -> (-7.8667, -58.0455) centre (0, -59.5) ccw projected
  arc A67 (-10.8167, -60.5) -> (-7.8667, -58.0455) centre (-10.8167, -57.5) ccw projected
  line L27 (-10.8167, -60.5) -> (-66.6833, -60.5) projected
  arc A68 (-10.8167, -62.3) -> (-6.0967, -58.3727) centre (-10.8167, -57.5) ccw
  line L28 (-10.8167, -62.3) -> (-66.6833, -62.3)
  arc A69 (-71.4033, -58.3727) -> (-66.6833, -62.3) centre (-66.6833, -57.5) ccw
  arc A70 (-71.4033, -58.3727) -> (-83.5967, -58.3727) centre (-77.5, -59.5) ccw
  arc A71 (-88.3167, -62.3) -> (-83.5967, -58.3727) centre (-88.3167, -57.5) ccw
  line L29 (-88.3167, -62.3) -> (-107.5, -62.3)
  arc A72 (-112.3, -57.5) -> (-107.5, -62.3) centre (-107.5, -57.5) ccw
  line L30 (-112.3, -57.5) -> (-112.3, -48.3167)
  arc A73 (-108.3727, -43.5967) -> (-112.3, -48.3167) centre (-107.5, -48.3167) ccw
  arc A74 (-108.3727, -43.5967) -> (-108.3727, -31.4033) centre (-109.5, -37.5) ccw
  arc A75 (-112.3, -26.6833) -> (-108.3727, -31.4033) centre (-107.5, -26.6833) ccw
  line L31 (-112.3, -26.6833) -> (-112.3, 26.6833)
  arc A76 (-108.3727, 31.4033) -> (-112.3, 26.6833) centre (-107.5, 26.6833) ccw
  arc A77 (-108.3727, 31.4033) -> (-108.3727, 43.5967) centre (-109.5, 37.5) ccw
  arc A78 (-112.3, 48.3167) -> (-108.3727, 43.5967) centre (-107.5, 48.3167) ccw
  line L32 (-112.3, 48.3167) -> (-112.3, 57.5)
  arc A79 (-107.5, 62.3) -> (-112.3, 57.5) centre (-107.5, 57.5) ccw
  line L33 (-107.5, 62.3) -> (-88.3167, 62.3)
  arc A80 (-83.5967, 58.3727) -> (-88.3167, 62.3) centre (-88.3167, 57.5) ccw
  arc A81 (-83.5967, 58.3727) -> (-71.4033, 58.3727) centre (-77.5, 59.5) ccw
  arc A82 (-66.6833, 62.3) -> (-71.4033, 58.3727) centre (-66.6833, 57.5) ccw
  line L34 (-66.6833, 62.3) -> (-10.8167, 62.3)
  arc A83 (-6.0967, 58.3727) -> (-10.8167, 62.3) centre (-10.8167, 57.5) ccw
  arc A84 (-6.0967, 58.3727) -> (6.0967, 58.3727) centre (0, 59.5) ccw
  arc A85 (10.8167, 62.3) -> (6.0967, 58.3727) centre (10.8167, 57.5) ccw
  line L35 (10.8167, 62.3) -> (66.6833, 62.3)
  arc A86 (71.4033, 58.3727) -> (66.6833, 62.3) centre (66.6833, 57.5) ccw
  arc A87 (71.4033, 58.3727) -> (83.5967, 58.3727) centre (77.5, 59.5) ccw
  arc A88 (88.3167, 62.3) -> (83.5967, 58.3727) centre (88.3167, 57.5) ccw
  line L36 (88.3167, 62.3) -> (107.5, 62.3)
  arc A89 (112.3, 57.5) -> (107.5, 62.3) centre (107.5, 57.5) ccw
  line L37 (112.3, 57.5) -> (112.3, 48.3167)
  arc A90 (108.3727, 43.5967) -> (112.3, 48.3167) centre (107.5, 48.3167) ccw
  arc A91 (108.3727, 43.5967) -> (108.3727, 31.4033) centre (109.5, 37.5) ccw
  arc A92 (112.3, 26.6833) -> (108.3727, 31.4033) centre (107.5, 26.6833) ccw
  line L38 (112.3, 26.6833) -> (112.3, -26.6833)
  arc A93 (108.3727, -31.4033) -> (112.3, -26.6833) centre (107.5, -26.6833) ccw
  arc A94 (108.3727, -31.4033) -> (108.3727, -43.5967) centre (109.5, -37.5) ccw
  arc A95 (112.3, -48.3167) -> (108.3727, -43.5967) centre (107.5, -48.3167) ccw
  line L39 (112.3, -48.3167) -> (112.3, -57.5)
  arc A96 (107.5, -62.3) -> (112.3, -57.5) centre (107.5, -57.5) ccw
  line L40 (107.5, -62.3) -> (88.3167, -62.3)
  arc A97 (83.5967, -58.3727) -> (88.3167, -62.3) centre (88.3167, -57.5) ccw
  arc A98 (83.5967, -58.3727) -> (71.4033, -58.3727) centre (77.5, -59.5) ccw
  arc A99 (66.6833, -62.3) -> (71.4033, -58.3727) centre (66.6833, -57.5) ccw
  line L41 (66.6833, -62.3) -> (10.8167, -62.3)
  arc A100 (6.0967, -58.3727) -> (10.8167, -62.3) centre (10.8167, -57.5) ccw
  arc A101 (6.0967, -58.3727) -> (-6.0967, -58.3727) centre (0, -59.5) ccw
  point P0 (0, 0)
  dimension "d106" = 0.2
  constraints: 68 point on circle, 34 centre point, 28 end point, 47 other
  measures "d106" radial gap between concentric circles of A20 A68
extrude "Extrusion7" cut sketch "Sketch7" against normal up to surface (5 mm away) contours A33 L13 A32 A31 A30 L12 A29 A28 A27 L11 A26 L10 A25 A24 A23 L9 A22 A21 A20 L8 A19 A18 A17 L7 A16 L6 A15 A14 A13 L5 A12 A11 A10 L4 A9 L3 A8 A7 A6 L2 A5 A4 A3 L1 A2 A1 A0 L0
chamfer "Chamfer5" distance 1 angle 45 48 edges at (7.7466, -61.1898, -59) (0, -53.3, -59) (-7.7466, -61.1898, -59) (-38.75, -62.3, -59) (-69.7534, -61.1898, -59) (-77.5, -53.3, -59) (-85.2466, -61.1898, -59) (-97.9083, -62.3, -59) (-110.8941, -60.8941, -59) (-112.3, -52.9083, -59) (-111.1898, -45.2466, -59) (-103.3, -37.5, -59) (-111.1898, -29.7534, -59) (-112.3, 0, -59) (-111.1898, 29.7534, -59) (-103.3, 37.5, -59) (-111.1898, 45.2466, -59) (-112.3, 52.9083, -59) (-110.8941, 60.8941, -59) (-97.9083, 62.3, -59) (-85.2466, 61.1898, -59) (-77.5, 53.3, -59) (-69.7534, 61.1898, -59) (-38.75, 62.3, -59) (-7.7466, 61.1898, -59) (0, 53.3, -59) (7.7466, 61.1898, -59) (38.75, 62.3, -59) (69.7534, 61.1898, -59) (77.5, 53.3, -59) (85.2466, 61.1898, -59) (97.9083, 62.3, -59) (110.8941, 60.8941, -59) (112.3, 52.9083, -59) (111.1898, 45.2466, -59) (103.3, 37.5, -59) (111.1898, 29.7534, -59) (112.3, 0, -59) (111.1898, -29.7534, -59) (103.3, -37.5, -59) (111.1898, -45.2466, -59) (112.3, -52.9083, -59) (110.8941, -60.8941, -59) (97.9083, -62.3, -59) (85.2466, -61.1898, -59) (77.5, -53.3, -59) (69.7534, -61.1898, -59) (38.75, -62.3, -59)
equation "\"d16\" = d17"
equation "\"d18\" = d17"
equation "\"d19\" = d17"
equation "\"d20\" = d17"
body "Solid1"
